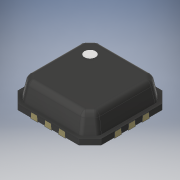
# Autodesk Inventor part: Semiconductor_QFN24-4x4
Saved by Autodesk Inventor 2018 (Build 220112000, 112)
## iProperties
Created: 2016-07-11
Part Number: Semiconductor_QFN24-4x4
Material: ABS Plastic
Document SubType Name: Modeling
Designer: Bradley
Density: 1.06 g/cm^3
Appearance: Smooth - Black
Author: Bradley
Autodesk Inventor part; units mm, degrees
ref_plane "YZ Plane" through (0, 0, 0) normal (1, 0, 0) x (0, 1, 0)
ref_plane "XZ Plane" through (0, 0, 0) normal (0, 1, 0) x (-1, 0, 0)
ref_plane "XY Plane" through (0, 0, 0) normal (0, 0, 1) x (1, 0, 0)
sketch "Sketch1" plane through (0, 0, 0) normal (0, 1, 0) x (-1, 0, 0)
  line L0 (-1.1, 1.5) -> (1.1, 1.5)
  line L1 (1.5, 1.1) -> (1.5, -1.1)
  line L2 (1.1, -1.5) -> (-1.1, -1.5)
  line L3 (-1.5, -1.1) -> (-1.5, 1.1)
  line L4 (-1.5, 1.5) -> (1.5, -1.5) construction
  line L5 (1.5, 1.5) -> (-1.5, -1.5) construction
  line L6 (1.5, 1.1) -> (1.1, 1.5)
  line L7 (-1.1, 1.5) -> (-1.5, 1.1)
  line L8 (-1.5, -1.1) -> (-1.1, -1.5)
  line L9 (1.1, -1.5) -> (1.5, -1.1)
  point P0 (0, 0)
  dimension "d0" = 3
  dimension "d1" = 3
  dimension "d68" = 0.4
  constraints: 20 end point, 8 point on line, 7 perpendicular, 2 midpoint, 2 parallel, 1 horizontal, 1 horizontal alignment
  measures "d0" distance of L4.end L5.end
  measures "d1" distance of L5.start L4.end
  measures "d68" distance of L1.start L5.start
extrude "Extrusion1" add sketch "Sketch1" along normal mid plane 0.2
sketch "Sketch2" plane through (0, -0.1, 0) normal (0, -1, 0) x (1, 0, 0)
  line L0 (0.75, 0.75) -> (-0.75, 0.75)
  line L1 (-0.75, 0.75) -> (-0.75, -0.75)
  line L2 (-0.75, -0.75) -> (0.75, -0.75)
  line L3 (0.75, -0.75) -> (0.75, 0.75)
  line L4 (0.75, 0.75) -> (-0.75, -0.75) construction
  line L5 (-0.75, 0.75) -> (0.75, -0.75) construction
  line L6 (1.1, 1.5) -> (-1.1, 1.5) projected
  line L7 (-1.5, 1.1) -> (-1.5, -1.1) projected
  line L8 (-1.1, -1.5) -> (1.1, -1.5) projected
  line L9 (1.5, -1.1) -> (1.5, 1.1) projected
  line L10 (0.625, -1.5) -> (0.375, -1.5)
  line L11 (0.375, -1.5) -> (0.375, -1.1)
  line L12 (0.375, -1.1) -> (0.625, -1.1)
  line L13 (0.625, -1.1) -> (0.625, -1.5)
  line L14 (1.5, -0.625) -> (1.1, -0.625)
  line L15 (1.1, -0.625) -> (1.1, -0.375)
  line L16 (1.1, -0.375) -> (1.5, -0.375)
  line L17 (1.5, -0.375) -> (1.5, -0.625)
  line L18 (0.625, 1.5) -> (0.375, 1.5)
  line L19 (0.375, 1.5) -> (0.375, 1.1)
  line L20 (0.375, 1.1) -> (0.625, 1.1)
  line L21 (0.625, 1.1) -> (0.625, 1.5)
  line L22 (-1.5, -0.625) -> (-1.1, -0.625)
  line L23 (-1.1, -0.625) -> (-1.1, -0.375)
  line L24 (-1.1, -0.375) -> (-1.5, -0.375)
  line L25 (-1.5, -0.375) -> (-1.5, -0.625)
  line L26 (1.5, -0.125) -> (1.1, -0.125)
  line L27 (1.1, -0.125) -> (1.1, 0.125)
  line L28 (1.1, 0.125) -> (1.5, 0.125)
  line L29 (1.5, 0.125) -> (1.5, -0.125)
  line L30 (-1.5, -0.125) -> (-1.1, -0.125)
  line L31 (-1.5, 0.125) -> (-1.5, -0.125)
  line L32 (-1.1, 0.125) -> (-1.5, 0.125)
  line L33 (-1.1, -0.125) -> (-1.1, 0.125)
  line L34 (1.5, 0.375) -> (1.1, 0.375)
  line L35 (1.1, 0.375) -> (1.1, 0.625)
  line L36 (1.1, 0.625) -> (1.5, 0.625)
  line L37 (1.5, 0.625) -> (1.5, 0.375)
  line L38 (-1.5, 0.375) -> (-1.1, 0.375)
  line L39 (-1.5, 0.625) -> (-1.5, 0.375)
  line L40 (-1.1, 0.625) -> (-1.5, 0.625)
  line L41 (-1.1, 0.375) -> (-1.1, 0.625)
  line L42 (0.125, -1.5) -> (-0.125, -1.5)
  line L43 (-0.125, -1.5) -> (-0.125, -1.1)
  line L44 (-0.125, -1.1) -> (0.125, -1.1)
  line L45 (0.125, -1.1) -> (0.125, -1.5)
  line L46 (-0.125, 1.1) -> (0.125, 1.1)
  line L47 (-0.125, 1.5) -> (-0.125, 1.1)
  line L48 (0.125, 1.5) -> (-0.125, 1.5)
  line L49 (0.125, 1.1) -> (0.125, 1.5)
  line L50 (-0.375, -1.5) -> (-0.625, -1.5)
  line L51 (-0.625, -1.5) -> (-0.625, -1.1)
  line L52 (-0.625, -1.1) -> (-0.375, -1.1)
  line L53 (-0.375, -1.1) -> (-0.375, -1.5)
  line L54 (-0.625, 1.1) -> (-0.375, 1.1)
  line L55 (-0.625, 1.5) -> (-0.625, 1.1)
  line L56 (-0.375, 1.5) -> (-0.625, 1.5)
  line L57 (-0.375, 1.1) -> (-0.375, 1.5)
  line L58 (-1.1, 1.5) -> (-1.5, 1.1) projected
  line L59 (-1.5, -1.1) -> (-1.1, -1.5) projected
  line L60 (1.1, -1.5) -> (1.5, -1.1) projected
  line L61 (1.5, 1.1) -> (1.1, 1.5) projected
  point P0 (0, 0)
  point P1 (-0.5, -1.1)
  point P2 (0, 0)
  point P3 (0, 0)
  point P4 (1.1, 0)
  point P5 (0, -1.1)
  dimension "d4" = 1.5
  dimension "d5" = 1.5
  dimension "d8" = 0.4
  dimension "d9" = 0.25
  dimension "d20" = 0.5
  dimension "d63" = 0.5
  constraints: 108 end point, 10 parallel, 7 midpoint, 6 equal length, 6 horizontal, 6 point on line, 5 perpendicular, 2 collinear, 1 horizontal alignment, 1 vertical, 1 vertical alignment, 64 other
  measures "d4" distance of L4.end L2.end
  measures "d5" distance of L2.end L0.start
  measures "d8" distance of L14.start L14.end
  measures "d9" distance of L14.end L15.end
  measures "d20" distance of L14.start L26.start
  measures "d63" distance of L10.start L42.start
extrude "Extrusion2" add sketch "Sketch2" along normal blind 0.02 contours L3 L2 L1 L0 | L21 L20 L19 L6 | L9 L34 L35 L36 | L49 L46 L47 L6 | L9 L26 L27 L28 | L57 L54 L55 L6 | L9 L14 L15 L16 | L40 L41 L38 L7 | L8 L11 L12 L13 | L32 L33 L30 L7 | L8 L43 L44 L45 | L24 L23 L22 L7 | L8 L51 L52 L53
sketch "Sketch3" plane through (-1.5, -0.1, 1.5) normal (-1, 0, 0) x (0, 0, 1)
  line L0 (-2.6, 0.2) -> (-0.4, 0.2) projected
  line L1 (-2.125, 0) -> (-2.125, -0.02) projected
  line L2 (-1.875, -0.02) -> (-2.125, -0.02) projected
  line L3 (-1.875, 0) -> (-1.875, -0.02) projected
  line L4 (-1.625, 0) -> (-1.875, 0) projected
  line L5 (-1.625, 0) -> (-1.625, -0.02) projected
  line L6 (-1.375, -0.02) -> (-1.625, -0.02) projected
  line L7 (-1.375, 0) -> (-1.375, -0.02) projected
  line L8 (-1.125, 0) -> (-1.375, 0) projected
  line L9 (-1.125, 0) -> (-1.125, -0.02) projected
  line L10 (-0.875, -0.02) -> (-1.125, -0.02) projected
  line L11 (-0.875, 0) -> (-0.875, -0.02) projected
  line L12 (-0.4, 0) -> (-0.875, 0) projected
  line L13 (-2.125, 0) -> (-1.875, 0) projected
  line L14 (-2.125, 0) -> (-2.1094, 0.183)
  line L15 (-2.1094, 0.183) -> (-1.8906, 0.183)
  line L16 (-1.8906, 0.183) -> (-1.875, 0)
  line L17 (-0.4, 0.2) -> (-0.4, 0) projected
  line L18 (-2.6, 0) -> (-2.6, 0.2) projected
  line L19 (-2.125, 0) -> (-2.6, 0) projected
  point P0 (-1.5, 0.1)
  dimension "d28" = 0.203
  dimension "d29" = 0.25
  dimension "d30" = 0.2188
  constraints: 6 end point, 1 equal length, 1 parallel
  measures "d28" distance between parallel lines of L2 L15
  measures "d29" distance of L2.start L1.end
  measures "d30" distance of L14.end L15.end
extrude "Extrusion3" add sketch "Sketch3" along normal blind 0.01 contours L13 L3 L2 L1 | L14 L15 L16 L13
pattern_linear "Rectangular Pattern1" count 3 spacing 0.5 along (0, 0, 1) of "Extrusion3"
pattern_circular "Circular Pattern1" count 4 over 360 about axis through (0, -10, 0) along (0, 1, 0) of "Extrusion3", "Rectangular Pattern1"
sketch "Sketch6" plane through (0, 0.1, 0) normal (0, 1, 0) x (1, 0, 0)
  line L0 (-1.5, -1.1) -> (-1.1, -1.5) projected
  line L1 (-1.1, -1.5) -> (1.1, -1.5) projected
  line L2 (1.1, -1.5) -> (1.5, -1.1) projected
  line L3 (1.5, -1.1) -> (1.5, 1.1) projected
  line L4 (1.5, 1.1) -> (1.1, 1.5) projected
  line L5 (1.1, 1.5) -> (-1.1, 1.5) projected
  line L6 (-1.1, 1.5) -> (-1.5, 1.1) projected
  line L7 (-1.5, 1.1) -> (-1.5, -1.1) projected
  line L8 (1.0482, 1.375) -> (1.375, 1.0482)
  line L9 (1.375, 1.0482) -> (1.375, -1.0482)
  line L10 (1.375, -1.0482) -> (1.0482, -1.375)
  line L11 (1.0482, -1.375) -> (-1.0482, -1.375)
  line L12 (-1.0482, -1.375) -> (-1.375, -1.0482)
  line L13 (-1.375, -1.0482) -> (-1.375, 1.0482)
  line L14 (-1.375, 1.0482) -> (-1.0482, 1.375)
  line L15 (-1.0482, 1.375) -> (1.0482, 1.375)
  point P0 (0, 0)
  dimension "d78" = 2.75
  constraints: 16 end point, 7 other
  measures "d78" distance between parallel lines of L13 L9
extrude "Extrusion6" add sketch "Sketch6" along normal blind 0.65 draft -12 contours L8 L9 L10 L11 L12 L13 L14 L15
fillet "Fillet1" radius 0.2 16 edges at (1.2368, 0.75, 0) (1.3059, 0.425, 1.0196) (1.3059, 0.425, -1.0196) (1.1139, 0.75, 1.1139) (1.0196, 0.425, 1.3059) (0, 0.75, 1.2368) (-1.0196, 0.425, 1.3059) (-1.1139, 0.75, 1.1139) (-1.3059, 0.425, 1.0196) (-1.2368, 0.75, 0) (-1.3059, 0.425, -1.0196) (-1.1139, 0.75, -1.1139) (-1.0196, 0.425, -1.3059) (0, 0.75, -1.2368) (1.0196, 0.425, -1.3059) (1.1139, 0.75, -1.1139)
sketch "Sketch7" plane through (0, 0.75, 0) normal (0, 1, 0) x (1, 0, 0)
  circle A0 centre (-0.6749, 0.6749) radius 0.2
  line L0 (-1.0749, -0.9239) -> (-1.0749, 0.9239) projected
  line L1 (-0.9239, -1.0749) -> (-1.0749, -0.9239) projected
  line L2 (0.9239, -1.0749) -> (-0.9239, -1.0749) projected
  line L3 (1.0749, -0.9239) -> (0.9239, -1.0749) projected
  line L4 (1.0749, 0.9239) -> (1.0749, -0.9239) projected
  line L5 (0.9239, 1.0749) -> (1.0749, 0.9239) projected
  line L6 (-0.9239, 1.0749) -> (0.9239, 1.0749) projected
  line L7 (-1.0749, 0.9239) -> (-0.9239, 1.0749) projected
  circle A1 centre (-0.6749, 0.6749) radius 0.4 construction
  line L8 (-0.9239, 1.0749) -> (0.9239, 1.0749) construction
  line L9 (-1.0749, -0.9239) -> (-1.0749, 0.9239) construction
  point P0 (0, 0)
  dimension "d82" = 0.4
  dimension "d83" = 0.2
  constraints: 2 centre point, 2 tangent, 1 coincident
  measures "d82" diameter of A0
  measures "d83" radial gap between concentric circles of A0 A1
extrude "Extrusion7" add sketch "Sketch7" along normal blind 0.01 contours A0
equation "\"d30\" = 0.875 * d29"
body "Solid1"
